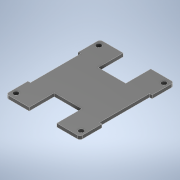
# Autodesk Inventor part: Placa de Aço
Saved by Autodesk Inventor 2021 (Build 250183000, 183)
## iProperties
Created: 2021-12-01
Part Number: Placa de Aço
Material: Genérico
Document SubType Name: Modeling
Designer: Administrador
Density: 8.73363 g/cm^3
Appearance: Padrão
Mass: 77.1 g
Surface Area: 77.3011 cm^2
Volume: 8.82795 cm^3
Author: Administrador
Autodesk Inventor part; units mm, degrees
ref_plane "YZ Plane" through (0, 0, 0) normal (1, 0, 0) x (0, 1, 0)
ref_plane "XZ Plane" through (0, 0, 0) normal (0, 1, 0) x (-1, 0, 0)
ref_plane "XY Plane" through (0, 0, 0) normal (0, 0, 1) x (1, 0, 0)
sketch "Esboço1" plane through (0, 0, 0) normal (0, 1, 0) x (-1, 0, 0)
  line L0 (-29.5, 35.5) -> (-29.5, 20)
  line L1 (-29.5, 20) -> (-27.5, 20)
  line L2 (-29.5, -35.5) -> (-29.5, -20)
  line L3 (-29.5, -20) -> (-27.5, -20)
  line L4 (-27.5, -20) -> (-27.5, 20)
  line L5 (29.5, 35.5) -> (29.5, 20)
  line L6 (29.5, 20) -> (27.5, 20)
  line L7 (29.5, -35.5) -> (29.5, -20)
  line L8 (29.5, -20) -> (27.5, -20)
  line L9 (27.5, -20) -> (27.5, 20)
  line L10 (-27.5, -37.5) -> (-11, -37.5)
  line L11 (-11, -37.5) -> (-11, -17.5)
  line L12 (27.5, -37.5) -> (11, -37.5)
  line L13 (11, -37.5) -> (11, -17.5)
  line L14 (11, -17.5) -> (-11, -17.5)
  line L15 (11, 37.5) -> (11, 17.5)
  line L16 (-27.5, 37.5) -> (-11, 37.5)
  line L17 (-11, 37.5) -> (-11, 17.5)
  line L18 (-11, 17.5) -> (11, 17.5)
  line L19 (27.5, 37.5) -> (11, 37.5)
  arc A0 (27.5, -37.5) -> (29.5, -35.5) centre (27.5, -35.5) ccw
  arc A1 (-29.5, -35.5) -> (-27.5, -37.5) centre (-27.5, -35.5) ccw
  arc A2 (-27.5, 37.5) -> (-29.5, 35.5) centre (-27.5, 35.5) ccw
  arc A3 (29.5, 35.5) -> (27.5, 37.5) centre (27.5, 35.5) ccw
  line L20 (0, -53.0799) -> (0, 53.0799) construction
  line L21 (-41.8799, 0) -> (41.8799, 0) construction
  line L22 (41.8799, 0) -> (-41.8799, 0) construction
  line L23 (0, -53.0799) -> (0, 53.0799) construction
  point P0 (0, 0)
  point P1 (29.5, -37.5)
  point P2 (29.5, 37.5)
  point P3 (-29.5, -37.5)
  dimension "d0" = 59
  dimension "d1" = 75
  dimension "d6" = 17.5
  dimension "d7" = 2
  dimension "d14" = 18.5
  dimension "d18" = 2
  dimension "d72" = 20
  dimension "d73" = 22
  constraints: 40 end point, 11 perpendicular, 8 point on circle, 8 tangent, 6 point on line, 6 vertical, 5 collinear, 5 equal length, 4 centre point, 4 parallel, 3 equal radius, 3 horizontal, 4 other
  measures "d0" distance of point (29.5, -37.5) point (-29.5, -37.5)
  measures "d1" distance of point (29.5, 37.5) point (29.5, -37.5)
  measures "d6" distance of point (29.5, 37.5) L5.end
  measures "d7" distance of L5.end L6.end
  measures "d14" distance of point (29.5, 37.5) L15.start
  measures "d18" radius of A0
  measures "d72" distance between parallel lines of L18 L19
  measures "d73" distance between parallel lines of L11 L13
extrude "Extrusão1" add sketch "Esboço1" along normal blind 2.65
sketch "Sketch7" plane through (0, 2.65, 0) normal (0, 1, 0) x (1, 0, 0)
  line L0 (27.5, 37.5) -> (11, 37.5) construction
  line L1 (29.5, 20) -> (29.5, 35.5) construction
  line L2 (-41.3, 0) -> (41.3, 0) construction
  line L3 (0, 52.5) -> (0, -52.5) construction
  point P0 (0, 0)
  point P1 (26, 33)
  point P2 (26, -33)
  point P3 (-26, -33)
  point P4 (-26, 33)
  dimension "d74" = 4.5
  dimension "d75" = 3.5
  constraints: 3 symmetric about line
  measures "d74" distance from line of L0 point (26, 33)
  measures "d75" distance from line of L1 point (26, 33)
hole "Hole5" at (26, 2.65, -33) at (26, 2.65, 33) at (-26, 2.65, 33) at (-26, 2.65, -33) direction (0, -1, 0) diameter 4 depth 2.65
